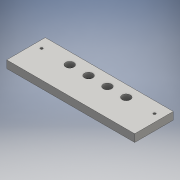
# Autodesk Inventor part: zStackJackAttach_piece1
Saved by Autodesk Inventor 2016 (Build 200138000, 138)
## iProperties
Created: 2016-10-04
Part Number: zStackJackAttach_piece1
Material: Generic
Document SubType Name: Modeling
Designer: sims01
Density: 1 g/cm^3
Appearance: Default
Author: sims01
Autodesk Inventor part; units mm, degrees
ref_plane "YZ Plane" through (0, 0, 0) normal (1, 0, 0) x (0, 1, 0)
ref_plane "XZ Plane" through (0, 0, 0) normal (0, 1, 0) x (-1, 0, 0)
ref_plane "XY Plane" through (0, 0, 0) normal (0, 0, 1) x (1, 0, 0)
sketch "Sketch1" plane through (0, 0, 0) normal (0, 0, 1) x (1, 0, 0)
  line L0 (-85, 15) -> (85, 15)
  line L1 (85, 15) -> (85, -15)
  line L2 (85, -15) -> (-85, -15)
  line L3 (-85, -15) -> (-85, 15)
  line L4 (85, -15) -> (-85, -15)
  line L5 (-85, -15) -> (-85, -36.3)
  line L6 (-85, -36.3) -> (85, -36.3)
  line L7 (85, -36.3) -> (85, -15)
  point P0 (0, 0)
  dimension "d0" = 30
  dimension "d1" = 170
  dimension "d2" = 85
  dimension "d3" = 15
  dimension "d34" = 21.3
  dimension "d35" = 170
  constraints: 16 end point, 4 parallel, 2 horizontal, 2 perpendicular
  measures "d0" distance of L2.end L0.start
  measures "d1" distance of L0.start L0.end
  measures "d2" distance from line of point (0, 0) L1
  measures "d3" distance from line of point (0, 0) L0
  measures "d34" distance of L4.end L5.end
  measures "d35" distance between parallel lines of L7 L5
extrude "Extrusion1" add sketch "Sketch1" along normal blind 10
sketch "Sketch2" plane through (0, 0, 10) normal (0, 0, 1) x (1, 0, 0)
  point P0 (0, 0)
  point P1 (-37.5, 0)
  point P2 (-12.5, 0)
  point P3 (12.5, 0)
  point P4 (37.5, 0)
  dimension "d30" = 25
  dimension "d31" = 25
  dimension "d32" = 25
  dimension "d33" = 12.5
  constraints: 4 horizontal alignment
  measures "d30" distance of point (-12.5, 0) point (-37.5, 0)
  measures "d31" distance of point (12.5, 0) point (-12.5, 0)
  measures "d32" distance of point (37.5, 0) point (12.5, 0)
  measures "d33" distance of point (0, 0) point (12.5, 0)
hole "Hole1" at (-37.5, 0, 10) at (-12.5, 0, 10) at (12.5, 0, 10) at (37.5, 0, 10) direction (0, 0, -1) diameter 6.6 end through all counterbore diameter 11 counterbore depth 7 clearance for "Hex Head Cap Screw ISO 24017" size "M6" standard "ISO"
sketch "Sketch3" plane through (0, 0, 10) normal (0, 0, 1) x (1, 0, 0)
  point P0 (0, 0)
  point P1 (75, 0)
  point P2 (-75, 0)
  dimension "d16" = 150
  dimension "d17" = 75
  constraints: 2 horizontal alignment
  measures "d16" distance of point (-75, 0) point (75, 0)
  measures "d17" distance of point (-75, 0) point (0, 0)
hole "Hole2" at (75, 0, 10) at (-75, 0, 10) direction (0, 0, -1) diameter 3.242 end through all thread size "M4x0.7" class "6H" standard "ISO Metric profile"
equation "\"d2\" = 0.5 * d1"
equation "\"d3\" = 0.5 * d0"
equation "\"d35\" = d1"
equation "\"d33\" = 0.5 * d31"
equation "\"d17\" = 0.5 * d16"
body "Solid1"
